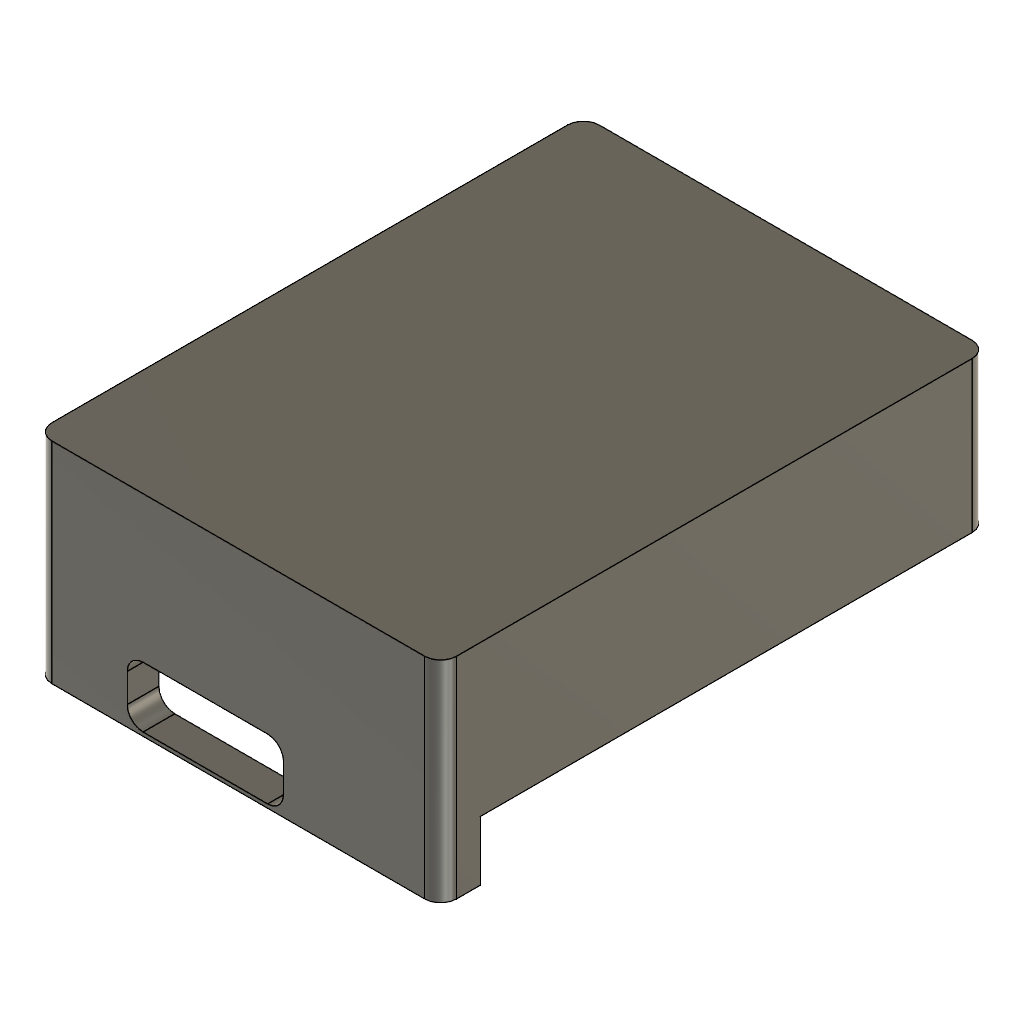
host bridge module (Autodesk Fusion 360 design; units mm, degrees)
description: KiCad electronic assembly
part number: empty 1
part number: PinHeader_2x07_P2.54mm_Horizontal
part number: R_0805_2012Metric
part number: empty_PCB
Autodesk Fusion 360 part; units mm, degrees
sketch "Sketch1" plane through (0, 0, 1.51) normal (0, 0, 1) x (-1, 0, 0) in component "Case"
  arc A0 (-12.75, -15) -> (-11.75, -16) centre (-11.75, -15) ccw
  line L0 (-11.75, -16) -> (11.75, -16)
  arc A1 (11.75, -16) -> (12.75, -15) centre (11.75, -15) ccw
  line L1 (12.75, -15) -> (12.75, 15)
  arc A2 (12.75, 15) -> (11.75, 16) centre (11.75, 15) ccw
  line L2 (11.75, 16) -> (-11.75, 16)
  arc A3 (-11.75, 16) -> (-12.75, 15) centre (-11.75, 15) ccw
  line L3 (-12.75, 15) -> (-12.75, -15)
  circle A4 centre (-5, 10.5) radius 1.1
  circle A5 centre (5, -2) radius 1.1
  circle A6 centre (7.64, -9.38) radius 0.5
  circle A7 centre (5.1, -9.38) radius 0.5
  circle A8 centre (7.64, -11.92) radius 0.5
  circle A9 centre (5.1, -11.92) radius 0.5
  circle A10 centre (2.56, -9.38) radius 0.5
  circle A11 centre (2.56, -11.92) radius 0.5
  circle A12 centre (0.02, -9.38) radius 0.5
  circle A13 centre (-2.52, -9.38) radius 0.5
  circle A14 centre (0.02, -11.92) radius 0.5
  circle A15 centre (-2.52, -11.92) radius 0.5
  circle A16 centre (-5.06, -9.38) radius 0.5
  circle A17 centre (-7.6, -9.38) radius 0.5
  circle A18 centre (-5.06, -11.92) radius 0.5
  circle A19 centre (-7.6, -11.92) radius 0.5
  line L4 (12.75, 18.5) -> (-12.75, 18.5)
  line L5 (-12.75, 18.5) -> (-12.75, -16)
  line L6 (-12.75, -16) -> (12.75, -16)
  line L7 (12.75, -16) -> (12.75, 18.5)
  dimension "d4" = 2.5
  constraint horizontal L4
  constraint vertical L5
  constraint horizontal L6
  constraint vertical L7
  constraint coincident L3 L4.end
  constraint coincident L1 L4.start
  constraint coincident L0 L6.end
  measures "d4" vertical distance of L2.end L4.end
extrude "Extrude1" add sketch "Sketch1" along normal blind 9.5 contours A0 L0 A1 L1 A2 L2 A3 L3 L5 L6 L7 | A2 L2 A3 L4 L5 L7 | A4 | A5 | A6 | A7 | A8 | A9 | A10 | A11 | A12 | A13 | A14 | A15 | A16 | A17 | A18 | A19 in component "Case"
shell "Shell1" thickness 2 removed faces 1 at (-4.25, -5, 1.51) in component "Case"
sketch "Sketch3" plane through (0, 0, 1.51) normal (0, 0, -1) x (1, 0, 0) in component "Case"
  line L0 (10.75, -14) -> (-10.75, -14)
  line L1 (-10.75, -14) -> (-10.75, 16.5)
  line L2 (-10.75, 16.5) -> (10.75, 16.5)
  line L3 (10.75, 16.5) -> (10.75, -14)
  arc A0 (-12.75, -15) -> (-11.75, -16) centre (-11.75, -15) ccw
  line L4 (-11.75, -16) -> (11.75, -16)
  arc A1 (11.75, -16) -> (12.75, -15) centre (11.75, -15) ccw
  line L5 (12.75, -15) -> (12.75, 18.5)
  line L6 (12.75, 18.5) -> (-12.75, 18.5)
  line L7 (-12.75, 18.5) -> (-12.75, -15)
  line L8 (-12.75, 16) -> (12.75, 16)
  line L9 (11.75, 16) -> (-11.75, 16)
  constraint coincident L7 L8.start
  constraint coincident L5 L8.end
  constraint perpendicular L5 L8
  constraint coincident L8.end L9
extrude "Extrude2" add sketch "Sketch3" along normal blind 3.75 contours L1 L2 L3 L5 L6 L7 L8 L9 in component "Case"
fillet "Fillet1" radius 1 2 edges at (-12.75, -18.5, 4.385) (12.75, -18.5, 4.385) in component "Case"
sketch "Sketch4" plane through (0, 16, 0) normal (0, 1, 0) x (-1, 0, 0) in component "Case"
  line L0 (-11.75, 1.51) -> (11.75, 1.51)
  line L1 (11.75, 1.51) -> (11.75, 11.01)
  line L2 (11.75, 11.01) -> (-11.75, 11.01)
  line L3 (-11.75, 11.01) -> (-11.75, 1.51)
  line L4 (-8.616, 6.675) -> (-6.584, 6.675)
  line L5 (-8.87, 1.849) -> (-8.87, 6.421)
  line L6 (8.91, 6.421) -> (8.91, 1.849)
  line L7 (-8.87, 6.675) -> (8.91, 6.675)
  line L8 (8.91, 6.675) -> (8.91, 1.51)
  line L9 (8.91, 1.51) -> (-8.87, 1.51)
  line L10 (-8.87, 1.51) -> (-8.87, 6.675)
  constraint horizontal L7
  constraint vertical L8
  constraint horizontal L9
  constraint vertical L10
  constraint coincident L4.end L7
  constraint coincident L5.end L10
  constraint coincident L6.start L8
  constraint coincident L0 L8.end
extrude "Extrude3" cut sketch "Sketch4" against normal up to surface (2 mm away) contours L0 L4 L5 L6 L7 L8 L9 L10 in component "Case"
move_face "OffsetFaces1" offset -0.4 3 faces at (2.9433, 15.3333, 6.675) (8.87, 15.3333, 3.2317) (-8.91, 15.3333, 4.9533) in component "Case"
chamfer "Chamfer1" distance 0.5 angle 45 2 edges at (9.27, 15, 7.075) (-9.31, 15, 7.075) in component "Case"
sketch "Sketch1 (2)" plane through (0, -18.5, 0) normal (0, -1, 0) x (1, 0, 0)
  line L0 (11.75, 20.76) -> (11.75, 34.01)
  line L1 (11.75, 34.01) -> (-11.75, 34.01)
  line L2 (-11.75, 34.01) -> (-11.75, 20.76)
  line L3 (-11.75, 20.76) -> (11.75, 20.76)
  line L4 (-6, 21) -> (1.8478, 21)
  line L5 (2.8478, 22) -> (2.8478, 23.8106)
  line L6 (1.8478, 24.8106) -> (-6, 24.8106)
  line L7 (-7, 23.8106) -> (-7, 22)
  arc A0 (2.8478, 23.8106) -> (1.8478, 24.8106) centre (1.8478, 23.8106) ccw
  arc A1 (1.8478, 21) -> (2.8478, 22) centre (1.8478, 22) ccw
  arc A2 (-6, 24.8106) -> (-7, 23.8106) centre (-6, 23.8106) ccw
  arc A3 (-7, 22) -> (-6, 21) centre (-6, 22) ccw
  dimension "d21" = 1
  constraint horizontal L4
  constraint vertical L5
  constraint horizontal L6
  constraint vertical L7
  constraint tangent L5 A0
  constraint tangent L6 A0
  constraint tangent L4 A1
  constraint tangent L5 A1
  constraint equal A0 A1
  constraint tangent L6 A2
  constraint tangent L7 A2
  constraint equal A0 A2
  constraint tangent L4 A3
  constraint tangent L7 A3
  constraint equal A0 A3
  measures "d21" radius of A0
extrude "Extrude4" cut sketch "Sketch1 (2)" against normal blind 4 contours L4 L5 L6 L7 A0 A1 A2 A3 sketch seen with x (1, 0, 0) y (0, 1, 0) z (0, 0, 1) at (0, 0, -23) in component "Case"
component "PinHeader_2x07_P2.54mm_Horizontal" placed x (0, 1, 0) y (-1, 0, 0) z (0, 0, 1) at (-7.64, 9.38, 1.595)
component "R_0805_2012Metric" placed x (1, 0, 0) y (0, 1, 0) z (0, 0, 1) at (-6.37, 6.0205, 1.595)
component "empty_PCB" placed x (1, 0, 0) y (0, 1, 0) z (0, 0, 1) at (0, 0, 0)
component "Case" placed x (1, 0, 0) y (0, 1, 0) z (0, 0, 1) at (0, 0, 23)
